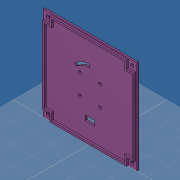
# Autodesk Inventor part: DayLightGlow_BaseCover
Saved by Autodesk Inventor 2019 (Build 230136000, 136)
## iProperties
Created: 2019-01-03
Part Number: DayLightGlow_BaseCover
Material: Generisch
Document SubType Name: Modeling
Designer: Stefan
Mass: 20.2009 g
Surface Area: 212.922 cm^2
Volume: 20.2009 cm^3
Density: 1 g/cm^3
Appearance: Glatt - Violett
Author: Stefan
Autodesk Inventor part; units mm, degrees
ref_plane "YZ Plane" through (0, 0, 0) normal (1, 0, 0) x (0, 1, 0)
ref_plane "XZ Plane" through (0, 0, 0) normal (0, 1, 0) x (-1, 0, 0)
ref_plane "XY Plane" through (0, 0, 0) normal (0, 0, 1) x (1, 0, 0)
sketch "Skizze1" plane through (0, 0, 0) normal (0, 0, 1) x (1, 0, 0)
  line L0 (48.8, -48.8) -> (-48.8, -48.8)
  line L1 (-48.8, -48.8) -> (-48.8, 48.8)
  line L2 (-48.8, 48.8) -> (48.8, 48.8)
  line L3 (48.8, 48.8) -> (48.8, -48.8)
  line L4 (48.8, -48.8) -> (-48.8, 48.8) construction
  line L5 (-48.8, -48.8) -> (48.8, 48.8) construction
  line L6 (-50, 50) -> (50, 50) construction
  line L7 (50, 50) -> (50, -50) construction
  line L8 (50, -50) -> (-50, -50) construction
  line L9 (-50, -50) -> (-50, 50) construction
  line L10 (-50, 50) -> (50, -50) construction
  line L11 (50, 50) -> (-50, -50) construction
  line L12 (-50, -50) -> (-40, -50) construction
  line L13 (-40, -50) -> (-40, -40) construction
  line L14 (-40, -40) -> (-50, -40) construction
  line L15 (-50, -40) -> (-50, -50) construction
  line L16 (50, -50) -> (40, -50) construction
  line L17 (40, -50) -> (40, -40) construction
  line L18 (40, -40) -> (50, -40) construction
  line L19 (50, -40) -> (50, -50) construction
  line L20 (50, 50) -> (40, 50) construction
  line L21 (40, 50) -> (40, 40) construction
  line L22 (40, 40) -> (50, 40) construction
  line L23 (50, 40) -> (50, 50) construction
  line L24 (-50, 50) -> (-40, 50) construction
  line L25 (-40, 50) -> (-40, 40) construction
  line L26 (-40, 40) -> (-50, 40) construction
  line L27 (-50, 40) -> (-50, 50) construction
  line L28 (47.75, -47.75) -> (-47.75, -47.75)
  line L29 (-47.75, -47.75) -> (-47.75, 47.75)
  line L30 (-47.75, 47.75) -> (47.75, 47.75)
  line L31 (47.75, 47.75) -> (47.75, -47.75)
  line L32 (47.75, -47.75) -> (-47.75, 47.75) construction
  line L33 (-47.75, -47.75) -> (47.75, 47.75) construction
  line L34 (-47.75, 40) -> (-45.75, 40)
  line L35 (-45.75, 40) -> (-45.75, -40)
  line L36 (-45.75, -40) -> (-47.75, -40)
  line L37 (-47.75, -40) -> (-47.75, 40)
  line L38 (-40, 47.75) -> (40, 47.75)
  line L39 (40, 47.75) -> (40, 45.75)
  line L40 (40, 45.75) -> (-40, 45.75)
  line L41 (-40, 45.75) -> (-40, 47.75)
  line L42 (47.75, 40) -> (45.75, 40)
  line L43 (45.75, 40) -> (45.75, -40)
  line L44 (45.75, -40) -> (47.75, -40)
  line L45 (47.75, -40) -> (47.75, 40)
  line L46 (40, -47.75) -> (-40, -47.75)
  line L47 (-40, -47.75) -> (-40, -45.75)
  line L48 (-40, -45.75) -> (40, -45.75)
  line L49 (40, -45.75) -> (40, -47.75)
  line L50 (-45.75, -38) -> (-38, -38)
  line L51 (-38, -38) -> (-38, -45.75)
  line L52 (45.75, -38) -> (38, -38)
  line L53 (38, -38) -> (38, -45.75)
  line L54 (38, 45.75) -> (38, 38)
  line L55 (38, 38) -> (45.75, 38)
  line L56 (-45.75, 38) -> (-38, 38)
  line L57 (-38, 38) -> (-38, 45.75)
  line L58 (40, 45.75) -> (40, 40)
  line L59 (45.75, 40) -> (40, 40)
  line L60 (38, 45.75) -> (40, 45.75)
  line L61 (45.75, 40) -> (45.75, 38)
  line L62 (38, -45.75) -> (40, -45.75)
  line L63 (40, -40) -> (40, -45.75)
  line L64 (40, -40) -> (45.75, -40)
  line L65 (45.75, -40) -> (45.75, -38)
  line L66 (-45.75, -40) -> (-40, -40)
  line L67 (-40, -45.75) -> (-40, -40)
  line L68 (-40, -45.75) -> (-38, -45.75)
  line L69 (-45.75, -40) -> (-45.75, -38)
  line L70 (-45.75, 38) -> (-45.75, 40)
  line L71 (-45.75, 40) -> (-40, 40)
  line L72 (-40, 40) -> (-40, 45.75)
  line L73 (-40, 45.75) -> (-38, 45.75)
  circle A0 centre (0, 0) radius 15 construction
  point P0 (0, 0)
  point P1 (0, 48.8)
  point P2 (44, 44)
  point P3 (-44, 44)
  point P4 (-44, -44)
  point P5 (44, -44)
  point P6 (0, 0)
  point P7 (-10.6066, 10.6066)
  point P8 (10.6066, 10.6066)
  point P9 (10.6066, -10.6066)
  point P10 (-10.6066, -10.6066)
  dimension "d0" = 97.6
  dimension "d1" = 97.6
  dimension "d27" = 100
  dimension "d28" = 100
  dimension "d29" = 10
  dimension "d30" = 4
  dimension "d40" = 95.5
  dimension "d41" = 2
  dimension "d42" = 2
  dimension "d55" = 30
  constraints: 148 end point, 35 point on line, 23 perpendicular, 22 parallel, 20 collinear, 13 midpoint, 12 horizontal, 4 point on circle, 3 equal length, 2 horizontal alignment, 2 vertical alignment, 1 centre point, 1 coincident, 1 vertical
  measures "d0" distance of L0.end L1.end
  measures "d1" distance of L1.end L2.end
  measures "d27" distance of L7.end L8.end
  measures "d28" distance of L6.end L7.end
  measures "d29" distance of L12.end L13.end
  measures "d30" distance from line of L13 point (-44, -44)
  measures "d40" distance of L29.end L30.end
  measures "d41" distance between parallel lines of L40 L30
  measures "d42" distance between parallel lines of L57 L25
  measures "d55" diameter of A0
extrude "Extrusion1" add sketch "Skizze1" against normal blind 2 contours L0 L1 L2 L3 | L28 L49 L63 L64 L44 L31 | L28 L47 L48 L49 | L44 L43 L42 L31 | L28 L29 L36 L66 L67 L47 | L48 L53 L52 L43 L64 L63 | L42 L59 L58 L39 L30 L31 | L67 L66 L35 L50 L51 L48 | L48 L51 L50 L35 L56 L57 L40 L54 L55 L43 L52 L53 | L43 L55 L54 L40 L58 L59 | L29 L34 L35 L36 | L39 L40 L41 L30 | L29 L30 L41 L72 L71 L34 | L71 L72 L40 L57 L56 L35
hole "Bohrung1" at (-44, -44, 0) at (44, -44, 0) at (44, 44, 0) at (-44, 44, 0) at (-10.6066, 10.6066, 0) at (10.6066, 10.6066, 0) at (-10.6066, -10.6066, 0) at (10.6066, -10.6066, 0) direction (0, 0, -1) diameter 3.4 end through all
extrude "Extrusion4" add sketch "Skizze1" along normal blind 2 contours L28 L47 L48 L49 | L44 L43 L42 L31 | L48 L53 L52 L43 L64 L63 | L67 L66 L35 L50 L51 L48 | L43 L55 L54 L40 L58 L59 | L29 L34 L35 L36 | L39 L40 L41 L30 | L71 L72 L40 L57 L56 L35
sketch "Skizze2" plane through (0, 0, -2) normal (0, 0, -1) x (-1, 0, 0)
  line L0 (-50, -50) -> (50, -50) construction
  line L1 (50, -50) -> (50, 50) construction
  line L2 (50, 50) -> (-50, 50) construction
  line L3 (-50, 50) -> (-50, -50) construction
  line L4 (-50, -50) -> (50, 50) construction
  line L5 (50, -50) -> (-50, 50) construction
  circle A0 centre (0, 0) radius 20 construction
  line L6 (0, 20) -> (0, 23)
  arc A1 (14.1421, 14.1421) -> (0, 20) centre (0, 0) ccw
  arc A2 (16.2635, 16.2635) -> (0, 23) centre (0, 0) ccw
  line L7 (14.1421, 14.1421) -> (16.2635, 16.2635)
  line L8 (-5, -25) -> (5, -25)
  line L9 (5, -25) -> (5, -30)
  line L10 (5, -30) -> (-5, -30)
  line L11 (-5, -30) -> (-5, -25)
  line L12 (-5, -25) -> (5, -30) construction
  line L13 (5, -25) -> (-5, -30) construction
  point P0 (0, 0)
  point P1 (0, 0)
  point P2 (0, -27.5)
  point P3 (0, -27.5)
  dimension "d1" = 97.6
  dimension "d27" = 100
  dimension "d45" = 100
  dimension "d46" = 100
  dimension "d47" = 40
  dimension "d53" = 3
  dimension "d54" = 45
  dimension "d57" = 10
  dimension "d58" = 5
  dimension "d59" = 25
  constraints: 28 end point, 7 midpoint, 6 point on circle, 4 parallel, 3 centre point, 3 concentric, 2 horizontal, 2 perpendicular, 2 vertical alignment, 1 coincident, 1 line through centre, 1 vertical
  measures "d45" distance of L1.end L2.end
  measures "d46" distance of L2.end L0.start
  measures "d47" diameter of A0
  measures "d53" radial gap between concentric circles of A0 A2
  measures "d54" angle of L7 L6
  measures "d57" distance between parallel lines of L9 L11
  measures "d58" distance between parallel lines of L10 L8
  measures "d59" distance from line of point (0, 0) L8
extrude "Extrusion5" cut sketch "Skizze2" against normal through all
equation "\"d1\" = d0"
equation "\"d42\" = d41"
